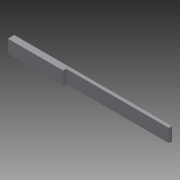
# Autodesk Inventor part: Bend Fix arm
Saved by Autodesk Inventor 2015 (Build 190159000, 159)
## iProperties
Created: 2017-12-31
Part Number: Bend Fix arm
Material: Generic
Document SubType Name: Modeling
Designer: Toby
Density: 1 g/cm^3
Appearance: Default
Author: Toby
Autodesk Inventor part; units mm, degrees
ref_plane "YZ Plane" through (0, 0, 0) normal (1, 0, 0) x (0, 1, 0)
ref_plane "XZ Plane" through (0, 0, 0) normal (0, 1, 0) x (-1, 0, 0)
ref_plane "XY Plane" through (0, 0, 0) normal (0, 0, 1) x (1, 0, 0)
sketch "Sketch1" plane through (0, 0, 0) normal (0, 0, 1) x (1, 0, 0)
  line L0 (-10.247, 2.4) -> (10.753, 2.4)
  line L1 (10.753, 2.4) -> (10.753, 0)
  line L2 (10.753, 0) -> (-10.247, 0)
  line L3 (-10.247, 0) -> (-10.247, 2.4)
  line L4 (10.753, 2.4) -> (49.753, 2.4)
  line L5 (49.753, 2.4) -> (49.753, 1.2)
  line L6 (49.753, 1.2) -> (10.753, 1.2)
  line L7 (10.753, 1.2) -> (10.753, 2.4)
  point P0 (0, 0)
  dimension "d0" = 2.4
  dimension "d1" = 1.2
  dimension "d2" = 60
  dimension "d3" = 21
  dimension "d4" = 1.2
  constraints: 16 end point, 4 parallel, 2 horizontal, 2 perpendicular
  measures "d0" distance of L2.end L0.start
  measures "d1" distance between parallel lines of L2 L6
  measures "d2" distance between parallel lines of L5 L3
  measures "d3" distance between parallel lines of L3 L1
  measures "d4" distance between parallel lines of L4 L6
extrude "Extrusion1" add sketch "Sketch1" along normal blind 5
body "Solid1"
